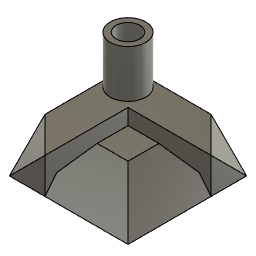
project 01 V.2 (Autodesk Fusion 360 design; units mm, degrees)
Autodesk Fusion 360 part; units mm, degrees
note: some values were not read from the file. Chosen so that the rebuilt part matches the saved one: that a step has no effect.
sketch "Sketch1" plane through (0, 0, 0) normal (0, 1, 0) x (1, 0, 0)
  line L0 (0, 0) -> (50, 0)
  line L1 (50, 0) -> (50, -50)
  line L2 (50, -50) -> (0, -50)
  line L3 (0, -50) -> (0, 0)
  line L4 (10, -49) -> (10, -50)
  line L5 (10, -49) -> (10, -10)
  line L6 (10, -10) -> (50, -10)
  line L7 (50, 0) -> (50, -10)
  line L8 (0, -50) -> (10, -50)
  line L9 (10, -50) -> (10, -10)
  dimension "d1" = 50
  dimension "d2" = 50
  constraint horizontal L0
  constraint vertical L1
  constraint horizontal L2
  constraint vertical L3
  constraint coincident L0.start L3.end
  constraint coincident L2 L4.end
  constraint perpendicular L2 L4
  constraint perpendicular L0 L5
  constraint coincident L1 L6.end
  constraint perpendicular L1 L6
  measures "d1" distance of L0.start L0.end
  measures "d2" distance of L0.start L2.end
sketch "Sketch2" plane through (0, 0, 0) normal (0, 1, 0) x (1, 0, 0)
sketch "Sketch4" plane through (0, 0, 0) normal (0, 1, 0) x (1, 0, 0)
  line L0 (10, -10) -> (50, -10)
  line L1 (50, -10) -> (50, -50)
  line L2 (50, -50) -> (10, -50)
  line L3 (10, -50) -> (10, -10)
  constraint horizontal L0
  constraint vertical L1
  constraint horizontal L2
  constraint vertical L3
extrude "Extrude5" add sketch "Sketch4" along normal blind 25
sketch "Sketch5" plane through (0, 25, 0) normal (0, 1, 0) x (-1, 0, 0)
  line L0 (-10, 50) -> (-50, 50)
  line L1 (-50, 50) -> (-50, 10)
  line L2 (-50, 10) -> (-10, 10)
  line L3 (-10, 10) -> (-10, 50)
  line L4 (-10, 10) -> (-50, 50)
  line L5 (-10, 50) -> (-50, 10)
  line L6 (-30, 30) -> (-10, 50)
  constraint coincident L2.end L3.start
  constraint coincident L0.end L1.start
  constraint coincident L0.start L3.end
  constraint coincident L1.end L2.start
  constraint midpoint L4 L6.start
sketch "Sketch7" plane through (0, 25, 0) normal (0, 1, 0) x (-1, 0, 0)
sketch "Sketch8" plane through (10, 0, 0) normal (-1, 0, 0) x (0, 0, 1)
  line L0 (50, 0) -> (50, 25)
  line L1 (50, 25) -> (10, 25)
  line L2 (10, 25) -> (10, 0)
  line L3 (10, 25) -> (10, 0)
  line L4 (50, 25) -> (50, 0)
  line L5 (10, 0) -> (50, 0)
  constraint coincident L1.end L2.start
  constraint coincident L0.end L1.start
sketch "Sketch9" plane through (50, 0, 0) normal (1, 0, 0) x (0, 0, -1)
  line L0 (-50, 0) -> (-10, 0)
  line L1 (-10, 0) -> (-10, 25)
  line L2 (-10, 25) -> (-50, 25)
  line L3 (-50, 25) -> (-50, 0)
  line L4 (-10, 25) -> (-10, 0)
  constraint coincident L1.end L2.start
  constraint coincident L0 L1.start
  constraint perpendicular L0 L4
sketch "Sketch10" plane through (0, 0, 50) normal (0, 0, 1) x (1, 0, 0)
  line L0 (10, 0) -> (50, 0)
  line L1 (50, 0) -> (50, 25)
  line L2 (50, 25) -> (10, 25)
  line L3 (10, 25) -> (10, 0)
  line L4 (10, 0, 0) -> (30, 25, -20)
  line L5 (30, 25, -20) -> (50, 0, 0)
  line L6 (30, 25, -20) -> (50, 0, -40)
  line L7 (50, 0, -40) -> (50, 0, 0)
  line L8 (30, 25, -20) -> (10, 0, -40)
  line L9 (10, 0, -40) -> (50, 0, -40)
  line L10 (30, 25, -20) -> (10, 0, -40)
  line L11 (10, 0, 0) -> (10, 0, -40)
  point P0 (10, 0)
  point P1 (30, 25)
  point P2 (50, 0)
  point P3 (10, 0)
  constraint coincident P3 P0
  constraint coincident L0.end L1.start
  constraint coincident P2 L0.end
sketch "Sketch10 (curves on the plane with normal 0, 0.6247, 0.7809 at 0 mm)" plane through (0, 0, 50) normal (0, 0.624695, 0.780869) x (-1, 0, 0)
  line L0 (-10, 0) -> (-50, 0)
  line L1 (-10, 0) -> (-30, -32.0156)
  line L2 (-30, -32.0156) -> (-50, 0)
extrude "Extrude6" cut sketch "Sketch10 (curves on the plane with normal 0, 0.6247, 0.7809 at 0 mm)" along normal blind 52
sketch "Sketch10 (curves on the plane with normal 0.7809, 0.6247, 0 at 39.0434 mm)" plane through (30.4878, 24.3902, 50) normal (0.780869, 0.624695, 0) x (-0.624695, 0.780869, 0)
  line L0 (0.7809, -20) -> (-31.2348, 0)
  line L1 (0.7809, -20) -> (-31.2348, -40)
  line L2 (-31.2348, -40) -> (-31.2348, 0)
extrude "Extrude7" cut sketch "Sketch10 (curves on the plane with normal 0.7809, 0.6247, 0 at 39.0434 mm)" along normal blind 61
extrude "Extrude8" cut 1 faces at (39.2683, 16.6667, 43.3333) along direction (0.848115, 0.413714, -0.330972) blind 30
extrude "Extrude9" cut 1 faces at (45.935, 16.6667, 48.7186) along direction (0.297467, 0.145106, 0.943641) blind 27
extrude "Extrude10" [no effect]
extrude "Extrude11" cut 1 faces at (20.7317, 16.6667, 43.3333) along direction (-0.848115, 0.413714, -0.330972) blind 46
extrude "Extrude12" cut 1 faces at (14.065, 16.6667, 48.7186) along direction (-0.297467, 0.145106, 0.943641) blind 38
sketch "Sketch10 (curves on the plane with normal 0.7809, -0.6247, 0 at 7.8087 mm)" plane through (6.0976, -4.878, 50) normal (0.780869, -0.624695, 0) x (0.624695, 0.780869, 0)
  line L0 (6.247, 0) -> (38.2626, -20)
  line L1 (38.2626, -20) -> (6.247, -40)
  line L2 (38.2626, -20) -> (6.247, -40)
  line L3 (6.247, 0) -> (6.247, -40)
extrude "Extrude13" cut sketch "Sketch10 (curves on the plane with normal 0.7809, -0.6247, 0 at 7.8087 mm)" against normal blind 58
extrude "Extrude14" cut 1 faces at (43.3333, 16.6667, 20.7317) along direction (-0.330972, 0.413714, -0.848115) blind 26
extrude "Extrude15" cut 1 faces at (16.6667, 16.6667, 20.7317) along direction (0.330972, 0.413714, -0.848115) blind 42
extrude "Extrude16" cut 1 faces at (48.7186, 16.6667, 14.065) along direction (0.943641, 0.145106, -0.297467) blind 29
extrude "Extrude17" cut 1 faces at (11.2814, 16.6667, 14.065) along direction (-0.943641, 0.145106, -0.297467) blind 32
sketch "Sketch10 (curves on the plane with normal 0, -0.6247, 0.7809 at -31.2348 mm)" plane through (0, 19.5122, 25.6098) normal (0, -0.624695, 0.780869) x (1, 0, 0)
  line L0 (30, 7.0278) -> (50, -24.9878)
  line L1 (30, 7.0278) -> (10, -24.9878)
  line L2 (10, -24.9878) -> (50, -24.9878)
  line L3 (30, 7.0278) -> (10, -24.9878)
extrude "Extrude18" cut sketch "Sketch10 (curves on the plane with normal 0, -0.6247, 0.7809 at -31.2348 mm)" against normal blind 66
sketch "Sketch11" plane through (0, 24.3902, 30.4878) normal (0, 0.624695, 0.780869) x (1, 0, 0)
  line L0 (30, 0.7809) -> (10, -31.2348)
  line L1 (10, -31.2348) -> (50, -31.2348)
  line L2 (50, -31.2348) -> (30, 0.7809)
sketch "Sketch12" plane through (0, 24.3902, 30.4878) normal (0, 0.624695, 0.780869) x (1, 0, 0)
  line L0 (23.5, -9.625) -> (36.5, -9.625)
  constraint horizontal L0
sketch "Sketch13" plane through (0, 24.3902, 30.4878) normal (0, 0.624695, 0.780869) x (1, 0, 0)
  line L0 (50, -6.247, -31.2348) -> (30, 0.7809, 0)
  line L1 (36.5, -9.625, 0) -> (36.5021, -1.5039, -10.1545)
  line L2 (36.5021, -1.5039, -10.1545) -> (23.5, -1.5039, -10.1545)
  line L3 (23.5, -1.5039, -10.1545) -> (23.5, -9.625, 0)
  line L4 (23.5, -9.625) -> (36.5, -9.625)
  point P0 (36.5, -9.625)
  point P1 (23.5, -9.625)
  constraint coincident P0 L4.end
  constraint coincident P1 L4.start
sketch "Sketch13 (curves on the plane with normal 0, 1, -0.0002 at -7.5168 mm)" plane through (0, 16.8735, 30.4889) normal (0, 1, -0.000152) x (-1, 0, 0)
  line L0 (-36.5, 6.0115) -> (-36.5021, -6.991)
  line L1 (-36.5021, -6.991) -> (-23.5, -6.991)
  line L2 (-23.5, -6.991) -> (-23.5, 6.0115)
  line L3 (-23.5, 6.0115) -> (-36.5, 6.0115)
extrude "Extrude19" cut sketch "Sketch13 (curves on the plane with normal 0, 1, -0.0002 at -7.5168 mm)" along normal blind 57
extrude "Extrude21" add sketch "Sketch1" along normal blind 10 contours L0 L1 L2 L3 L4 L5 L6 L7 L8 L9
extrude "Extrude25" add 1 faces at (10, 3.3333, 36.6667) along direction (1, 0, 0) blind 5
extrude "Extrude26" add 1 faces at (26.6667, 3.3333, 10) along direction (0, 0, 1) blind 5
extrude "Extrude27" add 1 faces at (5, 10, 21.6667) along direction (0, 1, 0) blind 5
sketch "Sketch14" plane through (0, 15, 0) normal (0, 1, 0) x (-1, 0, 0)
  line L0 (0, 0) -> (0, 50)
  line L1 (0, 50) -> (-15, 50)
  line L2 (-15, 50) -> (-15, 15)
  line L3 (-15, 15) -> (-50, 15)
  line L4 (-50, 15) -> (-50, 0)
  line L5 (-50, 0) -> (0, 0)
sketch "Sketch16" plane through (0, 15, 0) normal (0, 1, 0) x (-1, 0, 0)
  line L0 (-50, 0) -> (0, 0)
  line L1 (0, 0) -> (0, 50)
  line L2 (0, 50) -> (-15, 50)
  line L3 (-15, 50) -> (-15, 15)
  line L4 (-15, 15) -> (-50, 15)
  line L5 (-50, 15) -> (-50, 0)
  circle A0 centre (-7.5, 7.5) radius 7.5
  circle A1 centre (-7.5, 7.5) radius 5
  line L6 (0, 50) -> (-15, 50)
  line L7 (0, 50) -> (0, 35)
  line L8 (0, 35) -> (-15, 50)
  line L9 (-50, 0) -> (-50, 15)
  line L10 (-50, 0) -> (-35, 0)
  line L11 (-35, 0) -> (-50, 15)
  dimension "d64" = 15
  dimension "d65" = 15
  dimension "d66" = 15
  dimension "d67" = 15
  constraint tangent L1 A0
  constraint concentric A0 A1
  constraint coincident L1.end L2.start
  constraint coincident L2 L3.start
  constraint perpendicular L2 L7
  constraint coincident L0.start L5.end
  constraint perpendicular L0 L9
  constraint perpendicular L5 L10
  measures "d64" distance of L1.end L2.end
  measures "d65" distance of L1.end L7.end
  measures "d66" distance of L0.start L4.end
  measures "d67" distance of L0.start L10.end
extrude "Extrude32" add sketch "Sketch16" along normal blind 20 contours A0
sketch "Sketch17" plane through (0, 0, 0) normal (-1, 0, 0) x (0, 0, 1)
  line L0 (0, 0) -> (50, 0)
  line L1 (50, 0) -> (50, 15)
  line L2 (50, 15) -> (7.5, 15)
  line L3 (7.5, 15) -> (0, 15)
  line L4 (0, 15) -> (0, 0)
  line L5 (35, 15) -> (50, 0)
  line L6 (50, 15, -15) -> (50, 0, 0)
  line L7 (35, 15, 0) -> (50, 15, -15)
  line L8 (15, 15, -50) -> (0, 15, -35)
  line L9 (0, 15, -35) -> (0, 0, -50)
  line L10 (0, 0, -50) -> (15, 15, -50)
  point P0 (35, 15)
  point P1 (50, 15)
  point P2 (15, 15)
  point P3 (0, 15)
  constraint coincident P0 L5.start
  constraint coincident L0.end L1.start
  constraint coincident P1 L1.end
  constraint coincident P3 L3.end
  constraint coincident L0.start L4.end
sketch "Sketch17 (curves on the plane with normal -0.5774, -0.5774, 0.5774 at -28.8675 mm)" plane through (16.6667, 16.6667, -16.6667) normal (-0.57735, -0.57735, 0.57735) x (0, 0.707107, 0.707107)
  line L0 (21.2132, -40.8248) -> (10.6066, -22.4537)
  line L1 (10.6066, -22.4537) -> (0, -40.8248)
  line L2 (0, -40.8248) -> (21.2132, -40.8248)
extrude "Extrude33" cut sketch "Sketch17 (curves on the plane with normal -0.5774, -0.5774, 0.5774 at -28.8675 mm)" against normal blind 24
sketch "Sketch17 (curves on the plane with normal -0.5774, 0.5774, 0.5774 at 28.8675 mm)" plane through (-16.6667, 16.6667, 16.6667) normal (-0.57735, 0.57735, 0.57735) x (0, 0.707107, -0.707107)
  line L0 (-14.1421, -20.4124) -> (-35.3553, -20.4124)
  line L1 (-24.7487, -38.7836) -> (-35.3553, -20.4124)
  line L2 (-14.1421, -20.4124) -> (-24.7487, -38.7836)
extrude "Extrude34" cut sketch "Sketch17 (curves on the plane with normal -0.5774, 0.5774, 0.5774 at 28.8675 mm)" along normal blind 91
